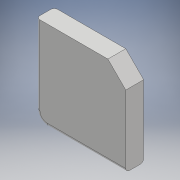
# Autodesk Inventor part: bearing bracket for bolt screw
Saved by Autodesk Inventor 2018 (Build 220112000, 112)
## iProperties
Created: 2018-04-10
Part Number: bearing bracket for bolt screw
Material: Generic
Document SubType Name: Modeling
Designer: m234676
Density: 1 g/cm^3
Appearance: Default
Author: m234676
Autodesk Inventor part; units mm, degrees
ref_plane "YZ Plane" through (0, 0, 0) normal (1, 0, 0) x (0, 1, 0)
ref_plane "XZ Plane" through (0, 0, 0) normal (0, 1, 0) x (-1, 0, 0)
ref_plane "XY Plane" through (0, 0, 0) normal (0, 0, 1) x (1, 0, 0)
sketch "Sketch2" plane through (0, 0, 0) normal (0, 1, 0) x (-1, 0, 0)
  line L0 (0, 0) -> (50, 0)
  line L1 (50, 0) -> (50, -50)
  line L2 (50, -50) -> (0, -50)
  line L3 (0, -50) -> (0, 0)
  dimension "d5" = 50
  dimension "d6" = 50
  constraints: 8 end point, 2 parallel, 1 horizontal, 1 perpendicular
  measures "d5" distance of L1.end L2.end
  measures "d6" distance of L0.end L1.end
extrude "Extrusion1" add sketch "Sketch2" along normal mid plane 10
sketch "Sketch3" plane through (0, 5, 0) normal (0, 1, 0) x (1, 0, 0)
  line L0 (-50, 0) -> (0, 0) construction
  line L1 (0, 0) -> (-31.8198, 31.8198) construction
  line L2 (0, 0) -> (45, 0) construction
  circle A0 centre (-31.8198, 31.8198) radius 12
  dimension "d9" = 45
  dimension "d10" = 135
  dimension "d11" = 24
  constraints: 4 end point, 1 centre point, 1 coincident, 1 equal length, 1 horizontal
  measures "d9" distance of L0.end L1.end
  measures "d10" angle of L2 L1
  measures "d11" diameter of A0
extrude "Extrusion2" cut sketch "Sketch3" against normal blind 2
chamfer "Chamfer1" distance 10 angle 45 1 edges at (0, 0, 0)
fillet "Fillet1" radius 6 1 edges at (-50, 0, -50)
fillet "Fillet1" radius 2 4 edges at (-25, 5, -50) (-25, -5, -50) (-50, -5, -25) (-50, 5, -25)
body "Solid1"
